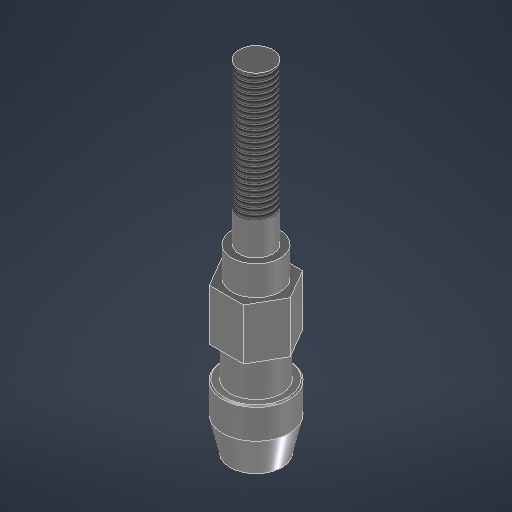
# Autodesk Inventor part: Soporte Bailarina
Saved by Autodesk Inventor 2026 (Build 300175000, 175)
## iProperties
Created: 2025-03-21
Part Number: Soporte Bailarina
Material: Steel, Alloy
Document SubType Name: Modeling
Designer: feder
Density: 7.73 g/cm^3
Appearance: Semi-Polished
Author: feder
Autodesk Inventor part; units mm, degrees
ref_plane "YZ Plane" through (0, 0, 0) normal (1, 0, 0) x (0, 1, 0)
ref_plane "XY Plane" through (0, 0, 0) normal (0, 0, 1) x (1, 0, 0)
sketch "Sketch1" plane through (0, 0, 0) normal (0, 1, 0) x (-1, 0, 0)
  circle A0 centre (0, 0) radius 9.7
  dimension "d0" = 19.4
  constraints: 1 centre point, 1 coincident
  measures "d0" diameter of A0
ref_plane "Work Plane1" through (0, 12.5, 0) normal (0, 1, 0) x (-1, 0, 0)
sketch "Sketch2" plane through (0, 12.5, 0) normal (0, 1, 0) x (-1, 0, 0)
  circle A0 centre (0, 0) radius 12.5
  dimension "d2" = 25
  constraints: 1 centre point, 1 coincident
  measures "d2" diameter of A0
loft "Loft1" add profiles "Sketch1", "Sketch2"
sketch "Sketch5" plane through (0, 12.5, 0) normal (0, 1, 0) x (1, 0, 0)
  circle A0 centre (0, 0) radius 12.5
  dimension "d9" = 25
  constraints: 1 centre point, 1 coincident
  measures "d9" diameter of A0
extrude "Extrusion1" add sketch "Sketch5" along normal blind 11.5
sketch "Sketch6" plane through (0, 24, 0) normal (0, 1, 0) x (1, 0, 0)
  circle A0 centre (0, 0) radius 9.65
  dimension "d12" = 19.3
  constraints: 1 centre point, 1 coincident
  measures "d12" diameter of A0
extrude "Extrusion2" add sketch "Sketch6" along normal blind 13.55
sketch "Sketch7" plane through (0, 37.55, 0) normal (0, 1, 0) x (1, 0, 0)
  line L0 (-6.3788, -11.1172) -> (-12.8171, -0.0344)
  line L1 (-12.8171, -0.0344) -> (-6.4384, 11.0828)
  line L2 (-6.4384, 11.0828) -> (6.3788, 11.1172)
  line L3 (6.3788, 11.1172) -> (12.8171, 0.0344)
  line L4 (12.8171, 0.0344) -> (6.4384, -11.0828)
  line L5 (6.4384, -11.0828) -> (-6.3788, -11.1172)
  point P0 (0, 0)
  point P1 (0, 0)
  dimension "d15" = 22.2
  constraints: 12 end point, 1 coincident, 13 other
  measures "d15" distance between parallel lines of L5 L2
extrude "Extrusion3" add sketch "Sketch7" along normal blind 19.15
sketch "Sketch8" plane through (0, 56.7, 0) normal (0, 1, 0) x (1, 0, 0)
  circle A0 centre (0, 0) radius 9.05
  dimension "d18" = 18.1
  constraints: 1 centre point, 1 coincident
  measures "d18" diameter of A0
extrude "Extrusion4" add sketch "Sketch8" along normal blind 11
sketch "Sketch9" plane through (0, 67.7, 0) normal (0, 1, 0) x (1, 0, 0)
  circle A0 centre (0, 0) radius 6.35
  dimension "d21" = 12.7
  constraints: 1 centre point, 1 coincident
  measures "d21" diameter of A0
extrude "Extrusion5" add sketch "Sketch9" along normal blind 14
sketch "Sketch10" plane through (0, 81.7, 0) normal (0, 1, 0) x (1, 0, 0)
  circle A0 centre (0, 0) radius 6.35
  dimension "d26" = 12.7
  constraints: 1 centre point, 1 coincident
  measures "d26" diameter of A0
extrude "Extrusion6" add sketch "Sketch10" along normal blind 46
thread "Thread2" size "1/2-13 UNC" class "2A" standard "ANSI Unified Screw Threads" length 48
chamfer "Chamfer1" distance 0.5 angle 45 1 edges at (-12.5, 24, 0)
body "Solid1"
